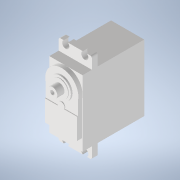
# Autodesk Inventor part: Motor Mg995
Saved by Autodesk Inventor 2022 (Build 260153000, 153)
## iProperties
Created: 2021-09-12
Part Number: Motor Mg995
Material: Generic
Document SubType Name: Modeling
Designer: Administrador
Density: 1 g/cm^3
Appearance: Default
Author: Administrador
Autodesk Inventor part; units mm, degrees
ref_plane "YZ Plane" through (0, 0, 0) normal (1, 0, 0) x (0, 1, 0)
ref_plane "XZ Plane" through (0, 0, 0) normal (0, 1, 0) x (-1, 0, 0)
ref_plane "XY Plane" through (0, 0, 0) normal (0, 0, 1) x (1, 0, 0)
sketch "Sketch1" plane through (0, 0, 0) normal (1, 0, 0) x (0, 1, 0)
  line L0 (0, 0) -> (0, 38) construction
  line L1 (7, 0) -> (47, 0)
  line L2 (0, 0) -> (7, 0)
  line L3 (7, 0) -> (47, 0)
  line L4 (47, 0) -> (47, 28)
  line L5 (7, 28) -> (7, 0)
  line L6 (47, 28) -> (54, 28) construction
  line L7 (54, 0) -> (54, 47.2) construction
  line L8 (54, 47.2) -> (0, 47.2) construction
  line L9 (0, 28) -> (0, 31.6)
  line L10 (54, 31.6) -> (54, 28)
  line L11 (7, 31.6) -> (7, 37.25)
  line L12 (7, 37.25) -> (47, 37.25)
  line L13 (47, 37.25) -> (47, 31.6)
  line L14 (0, 31.6) -> (7, 31.6)
  line L15 (47, 31.6) -> (54, 31.6)
  line L16 (54, 28) -> (47, 28)
  line L17 (7, 28) -> (0, 28)
  dimension "d0" = 38
  dimension "d1" = 54
  dimension "d3" = 40
  dimension "d4" = 28
  dimension "d5" = 47.2
  dimension "d6" = 3.6
  dimension "d7" = 5.65
  dimension "d49" = 28
  dimension "d50" = 5.65
  dimension "d51" = 3.6
  constraints: 36 end point, 8 perpendicular, 5 parallel, 3 horizontal, 3 vertical, 1 point on line
  measures "d0" distance of L0.start L0.end
  measures "d1" distance of L0.start L7.start
  measures "d3" distance of L1.start L1.end
  measures "d4" distance of L1.end L4.end
  measures "d5" distance of L7.start L7.end
  measures "d6" distance of L9.start L9.end
  measures "d7" distance of L11.start L11.end
  measures "d49" distance between parallel lines of L2 L17
  measures "d50" distance between parallel lines of L12 L15
  measures "d51" distance of L13.end L4.end
extrude "Extrusion1" add sketch "Sketch1" along normal blind 20
sketch "Sketch2" plane through (0, 7, 37.25) normal (0, 0, 1) x (1, 0, 0)
  line L0 (0, 40) -> (0, 0) projected
  line L1 (0, 0) -> (20, 0) projected
  line L2 (20, 40) -> (20, 0) projected
  line L3 (0, 40) -> (20, 40) projected
  line L4 (10, 39.7) -> (10, 30)
  line L5 (0, 0) -> (0, 40) projected
  circle A0 centre (10, 30) radius 1.3
  circle A1 centre (10, 30) radius 3
  arc A2 (19.7, 27.569) -> (0.3, 27.569) centre (10, 30) ccw
  line L6 (19.7, 27.569) -> (19.7, 6.969)
  line L7 (0.3, 6.969) -> (0.3, 27.569)
  arc A3 (5.5, 6.969) -> (14.5, 6.969) centre (10, 11.0315) ccw
  line L8 (19.7, 6.969) -> (14.5, 6.969)
  line L9 (5.5, 6.969) -> (0.3, 6.969)
  line L10 (10, 6.969) -> (10, 4.969) construction
  point P0 (0, -7)
  dimension "d11" = 9.7
  dimension "d12" = 2.6
  dimension "d13" = 6
  dimension "d14" = 20.6
  dimension "d19" = 9
  dimension "d20" = 2
  constraints: 12 end point, 5 point on circle, 4 centre point, 3 coincident, 1 parallel
  measures "d11" distance of L4.start L4.end
  measures "d12" diameter of A0
  measures "d13" diameter of A1
  measures "d14" distance of L6.start L6.end
  measures "d19" distance of L9.start L8.end
  measures "d20" distance of L10.start L10.end
extrude "Extrusion2" add sketch "Sketch2" along normal blind 2.5 contours A2 L6 L8 A3 L9 L7 | A0 | A1
sketch "Sketch3" plane through (0, 7, 39.75) normal (0, 0, 1) x (1, 0, 0)
  line L0 (14.5, 6.969) -> (19.7, 6.969) projected
  line L1 (0.3, 6.969) -> (0.3, 27.569) projected
  line L2 (19.7, 6.969) -> (0.3, 6.969)
  line L3 (0.3, 6.969) -> (0.3, 19.669)
  line L4 (19.7, 19.669) -> (19.7, 6.969)
  arc A0 (11.875, 19.669) -> (8.125, 19.669) centre (10, 20.6147) ccw
  line L5 (8.125, 19.669) -> (0.3, 19.669)
  line L6 (11.875, 19.669) -> (19.7, 19.669)
  point P0 (0, -7)
  dimension "d21" = 12.7
  dimension "d25" = 2.1
  dimension "d26" = 3.75
  constraints: 10 end point, 2 horizontal, 2 point on circle, 1 centre point, 1 parallel, 1 perpendicular, 1 point on line
  measures "d21" distance of L2.end L3.end
  measures "d25" radius of A0
  measures "d26" distance of L6.start L5.start
extrude "Extrusion3" add sketch "Sketch3" along normal blind 0.5
sketch "Sketch4" plane through (0, 7, 39.75) normal (0, 0, 1) x (1, 0, 0)
  line L0 (11.875, 19.669) -> (19.7, 19.669) projected
  line L1 (19.7, 19.669) -> (19.7, 27.569) projected
  arc A0 (19.7, 27.569) -> (0.3, 27.569) centre (10, 30) ccw projected
  line L2 (0.3, 27.569) -> (0.3, 19.669) projected
  line L3 (0.3, 19.669) -> (8.125, 19.669) projected
  arc A1 (11.875, 19.669) -> (8.125, 19.669) centre (10, 20.6147) ccw projected
  circle A2 centre (10, 30) radius 6.5
  point P0 (0, -7)
  dimension "d29" = 13
  constraints: 1 centre point, 1 coincident
  measures "d29" diameter of A2
extrude "Extrusion4" add sketch "Sketch4" along normal blind 1 contours A2
sketch "Sketch5" plane through (10, 37, 40.75) normal (0, 0, 1) x (1, 0, 0)
  circle A0 centre (0, 0) radius 5.25
  point P0 (-10, -37)
  dimension "d32" = 10.5
  constraints: 1 centre point
  measures "d32" diameter of A0
extrude "Extrusion5" add sketch "Sketch5" along normal blind 0.4
sketch "Sketch6" plane through (10, 37, 41.15) normal (0, 0, 1) x (1, 0, 0)
  circle A0 centre (0, 0) radius 3
  circle A1 centre (0, 0) radius 1.3
  point P0 (-10, -37)
  dimension "d35" = 6
  dimension "d36" = 2.6
  constraints: 2 centre point, 1 coincident
  measures "d35" diameter of A0
  measures "d36" diameter of A1
extrude "Extrusion6" add sketch "Sketch6" along normal blind 4.3
sketch "Sketch7" plane through (0, 0, 31.6) normal (0, 0, 1) x (1, 0, 0)
  line L0 (0, 7) -> (0, 0) projected
  line L1 (0, 0) -> (20, 0) projected
  line L2 (20, 7) -> (20, 0) projected
  line L3 (0, 7) -> (20, 7) projected
  line L4 (0, 54) -> (0, 47) projected
  line L5 (0, 47) -> (20, 47) projected
  line L6 (20, 54) -> (20, 47) projected
  line L7 (0, 54) -> (20, 54) projected
  line L8 (0, 0) -> (3, 0)
  arc A0 (5.5, 0) -> (3, 0) centre (4.25, 1.7493) ccw
  line L9 (10, 0) -> (10, 5.7084)
  arc A1 (17, 0) -> (14.5, 0) centre (15.75, 1.7493) ccw
  line L10 (17, 0) -> (14.5, 0)
  line L11 (0, 7) -> (0, 47) projected
  line L12 (0, 27) -> (24.9803, 27)
  line L13 (0, 54) -> (20, 54)
  line L14 (0, 54) -> (20, 54)
  line L15 (3, 54) -> (5.5, 54)
  arc A2 (3, 54) -> (5.5, 54) centre (4.25, 52.2507) ccw
  arc A3 (14.5, 54) -> (17, 54) centre (15.75, 52.2507) ccw
  line L16 (17, 54) -> (14.5, 54)
  line L17 (5.5, 54) -> (3, 54)
  line L18 (0, 54) -> (20, 54) projected
  line L19 (5.5, 0) -> (3, 0)
  point P0 (14.5, 54)
  point P1 (5.5, 54)
  point P2 (3, 54)
  point P3 (17, 0)
  point P4 (14.5, 0)
  point P5 (5.5, 0)
  point P6 (3, 0)
  dimension "d39" = 3
  dimension "d40" = 2.5
  dimension "d42" = 2.15
  dimension "d44" = 2.5
  dimension "d45" = 2.15
  constraints: 20 end point, 8 point on circle, 8 symmetric about line, 4 centre point, 3 collinear, 2 point on line, 1 horizontal, 1 midpoint, 1 vertical, 2 other
  measures "d39" distance of L8.start L8.end
  measures "d40" distance of L8.end L19.start
  measures "d42" radius of A0
  measures "d44" distance of L10.end L10.start
  measures "d45" radius of A1
extrude "Extrusion7" cut sketch "Sketch7" against normal up to surface (3.6 mm away) contours A0 L1 | L1 A1 | L7 A2 | L7 A3
fillet "Fillet1" radius 1 4 edges at (0, 0, 29.8) (20, 0, 29.8) (0, 54, 29.8) (20, 54, 29.8)
body "Solid1"
